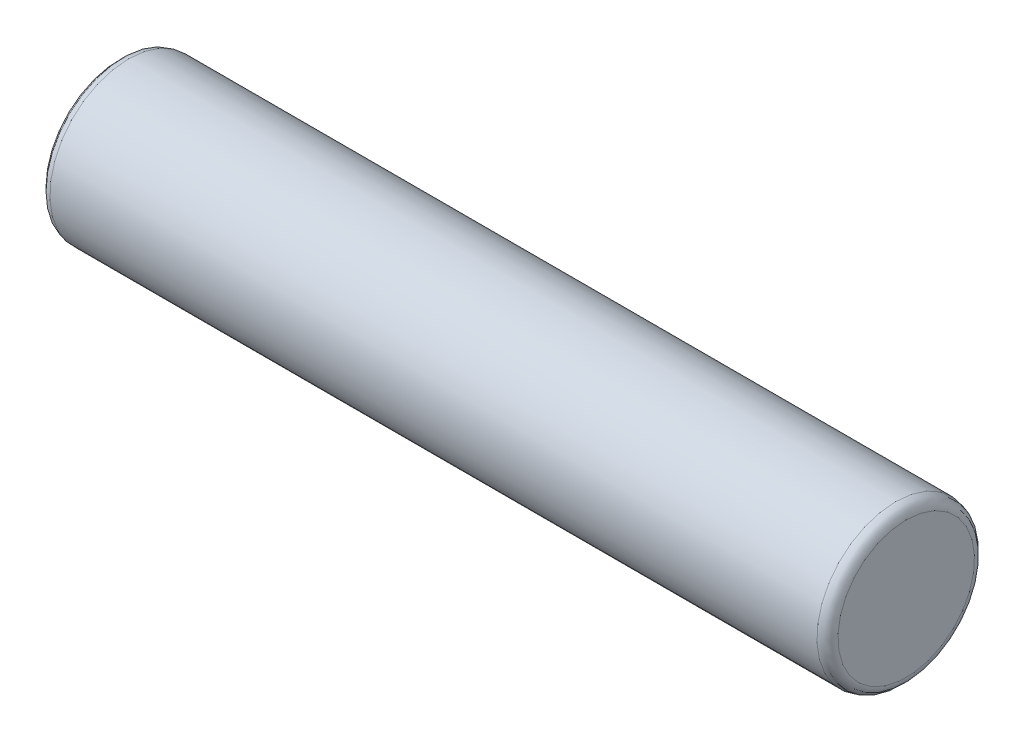
# Autodesk Inventor part: Lank
Saved by Autodesk Inventor 2026 (Build 300175000, 175)
## iProperties
Created: 2025-04-29
Part Number: Lank
Material: Generic
Document SubType Name: Modeling
Designer: elias
Density: 1 g/cm^3
Appearance: Default
Author: elias
Autodesk Inventor part; units mm, degrees
ref_plane "YZ Plane" through (0, 0, 0) normal (1, 0, 0) x (0, 1, 0)
ref_plane "XZ Plane" through (0, 0, 0) normal (0, 1, 0) x (-1, 0, 0)
ref_plane "XY Plane" through (0, 0, 0) normal (0, 0, 1) x (1, 0, 0)
sketch "Sketch1" plane through (0, 0, 0) normal (1, 0, 0) x (0, 1, 0)
  line L0 (3056.2025, 0) -> (3056.2025, -6694.5386) construction
  line L1 (3056.2025, -6694.5386) -> (0, -6694.5386) construction
  line L2 (0, -6694.5386) -> (0, 0) construction
  line L3 (0, 0) -> (3056.2025, 0) construction
  point P0 (0, 0)
  dimension "d15" = 150
  dimension "d16" = 0
  constraints: 2 end point, 2 other
sketch "Sketch2" plane through (0, 0, 0) normal (1, 0, 0) x (0, 1, 0)
  point P0 (0, 0)
sketch "Sketch3" plane through (0, 0, 0) normal (1, 0, 0) x (0, 1, 0)
  circle A0 centre (552.1662, -2872.1219) radius 15
  point P0 (0, 0)
  dimension "d14" = 30
  constraints: 1 centre point
  measures "d14" diameter of A0
extrude "Extrusion1" add sketch "Sketch3" along normal blind 150
fillet "Fillet1" radius 2 2 edges at (150, 537.1662, -2872.1219) (0, 537.1662, -2872.1219)
body "Solid1"
